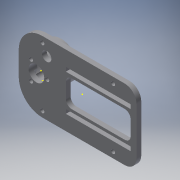
# Autodesk Inventor part: Slip_Plate_2bearing
Saved by Autodesk Inventor 2016 (Build 200138000, 138)
## iProperties
Created: 2015-10-15
Part Number: Slip_Plate_2bearing
Material: Generic
Document SubType Name: Modeling
Designer: USER
Density: 1 g/cm^3
Appearance: Default
Mass: 21.5255 g
Surface Area: 145.686 cm^2
Volume: 21.5255 cm^3
Author: USER
Autodesk Inventor part; units mm, degrees
ref_plane "YZ Plane" through (0, 0, 0) normal (1, 0, 0) x (0, 1, 0)
ref_plane "XZ Plane" through (0, 0, 0) normal (0, 1, 0) x (-1, 0, 0)
ref_plane "XY Plane" through (0, 0, 0) normal (0, 0, 1) x (1, 0, 0)
sketch "Sketch1" plane through (0, 0, 0) normal (0, 1, 0) x (-1, 0, 0)
  line L0 (-50, 30) -> (50, 30)
  line L1 (50, 30) -> (50, -30)
  line L2 (50, -30) -> (-50, -30)
  line L3 (-50, -30) -> (-50, 30)
  line L4 (0, 0) -> (0, 16.4238) construction
  line L5 (0, 0) -> (26.4574, 0) construction
  dimension "d0" = 100
  dimension "d1" = 60
  constraints: 12 end point, 3 parallel, 2 perpendicular, 1 horizontal, 2 other
  measures "d0" distance of L0.start L0.end
  measures "d1" distance of L0.end L1.end
extrude "Extrusion1" add sketch "Sketch1" along normal blind 4
sketch "Sketch2" plane through (0, 4, 0) normal (0, 1, 0) x (1, 0, 0)
  line L0 (50, -30) -> (50, 30) projected
  line L1 (-10, 17.25) -> (45, 17.25)
  line L2 (45, 17.25) -> (45, 13.75)
  line L3 (45, 13.75) -> (-10, 13.75)
  line L4 (-10, 13.75) -> (-10, 17.25)
  line L5 (-10, -13.75) -> (45, -13.75)
  line L6 (45, -13.75) -> (45, -17.25)
  line L7 (45, -17.25) -> (-10, -17.25)
  line L8 (-10, -17.25) -> (-10, -13.75)
  line L9 (0, 0) -> (41.7, 0) construction
  line L10 (-10, 15.5) -> (45, 15.5) construction
  line L11 (-10, -15.5) -> (45, -15.5) construction
  dimension "d4" = 3.5
  dimension "d5" = 31
  dimension "d6" = 5
  dimension "d7" = 55
  constraints: 22 end point, 4 midpoint, 4 parallel, 3 perpendicular, 2 horizontal, 4 other
  measures "d4" distance between parallel lines of L1 L3
  measures "d5" distance between parallel lines of L10 L11
  measures "d6" distance between parallel lines of L0 L2
  measures "d7" distance of L1.start L1.end
extrude "Extrusion2" cut sketch "Sketch2" against normal through all
sketch "Sketch3" plane through (0, 4, 0) normal (0, 1, 0) x (1, 0, 0)
  line L0 (-50, 30) -> (-50, -30) projected
  circle A0 centre (-35, 0) radius 6.65
  circle A1 centre (-25.79, 0) radius 1.7
  circle A2 centre (-39.605, 7.9761) radius 1.7
  circle A3 centre (-39.605, -7.9761) radius 1.7
  line L1 (-35, 0) -> (0, 0) construction
  line L2 (-35, 0) -> (-41.2469, 10.8199) construction
  line L3 (-35, 0) -> (-41.9983, -12.1214) construction
  circle A4 centre (-35, 0) radius 9.21 construction
  dimension "d10" = 120
  dimension "d11" = 120
  dimension "d12" = 18.42
  dimension "d13" = 13.3
  dimension "d14" = 3.4
  dimension "d15" = 3.4
  dimension "d16" = 3.4
  dimension "d17" = 15
  constraints: 6 end point, 5 centre point, 3 point on circle, 3 point on line, 1 coincident, 1 perpendicular
  measures "d10" angle of L2 L1
  measures "d11" angle of L3 L1
  measures "d12" diameter of A4
  measures "d13" diameter of A0
  measures "d14" diameter of A2
  measures "d15" diameter of A1
  measures "d16" diameter of A3
  measures "d17" distance from line of L0 L1.start
extrude "Extrusion3" cut sketch "Sketch3" against normal through all
sketch "Sketch4" plane through (0, 0, 0) normal (0, -1, 0) x (1, 0, 0)
  circle A0 centre (-35, 0) radius 6.65 projected
  line L0 (-10, 11.35) -> (45, 11.35)
  line L1 (45, 11.35) -> (45, -11.35)
  line L2 (45, -11.35) -> (-10, -11.35)
  line L3 (-10, -11.35) -> (-10, 11.35)
  line L4 (0, 0) -> (34.3745, 0) construction
  dimension "d20" = 25
  dimension "d21" = 55
  dimension "d22" = 22.7
  constraints: 10 end point, 2 parallel, 2 perpendicular, 1 horizontal, 1 other
  measures "d20" distance from line of L3 A0.centre
  measures "d21" distance of L0.start L0.end
  measures "d22" distance of L0.end L1.end
extrude "Extrusion4" cut sketch "Sketch4" against normal through all contours L0 L1 L2 L3
fillet "Fillet1" radius 10 2 edges at (50, 2, -30) (50, 2, 30)
fillet "Fillet2" radius 20 2 edges at (-50, 2, -30) (-50, 2, 30)
sketch "Sketch5" plane through (0, 0, 0) normal (0, -1, 0) x (1, 0, 0)
  line L0 (-50, 10) -> (-50, -10) projected
  line L1 (50, -20) -> (50, 20) projected
  line L2 (40, 30) -> (-30, 30) projected
  line L3 (-32.9422, 25) -> (22.0212, 25) construction
  line L4 (-20.947, -25) -> (23.6325, -25) construction
  line L5 (0, 0) -> (19.8728, 0) construction
  circle A0 centre (30, 25) radius 1.75
  circle A1 centre (-30, 25) radius 1.75
  circle A2 centre (-30, -25) radius 1.75
  circle A3 centre (30, -25) radius 1.75
  dimension "d27" = 5
  dimension "d28" = 3.5
  dimension "d29" = 3.5
  dimension "d30" = 20
  dimension "d31" = 20
  constraints: 6 end point, 4 centre point, 4 point on line, 3 parallel, 3 other
  measures "d27" distance between parallel lines of L2 L3
  measures "d28" diameter of A0
  measures "d29" diameter of A1
  measures "d30" distance from line of L0 A1.centre
  measures "d31" distance from line of L1 A0.centre
extrude "Extrusion5" cut sketch "Sketch5" against normal through all
fillet "Fillet3" radius 5 4 edges at (-10, 2, 11.35) (45, 2, 11.35) (45, 2, -11.35) (-10, 2, -11.35)
sketch "Sketch6" plane through (0, 4, 0) normal (0, 1, 0) x (1, 0, 0)
  circle A0 centre (-35, 0) radius 6.65 projected
  circle A1 centre (-35, 0) radius 11
  circle A2 centre (-35, 0) radius 6.65
  circle A3 centre (-35, 0) radius 15
  arc A4 (-24.3217, -2.6407) -> (-24.4212, 3.0147) centre (-26.9384, 0.1419) ccw
  arc A5 (-43.0674, -7.4777) -> (-37.985, -10.5872) centre (-39.1841, -6.8388) ccw
  arc A6 (-38.3451, 10.479) -> (-42.7646, 7.7917) centre (-39.7175, 7.7583) ccw
  point P0 (0, 0)
  dimension "d35" = 22
  constraints: 12 point on circle, 6 centre point, 3 coincident
  measures "d35" diameter of A1
extrude "Extrusion6" add sketch "Sketch6" along normal blind 17 contours A3
sketch "Sketch7" plane through (0, 4, 0) normal (0, 1, 0) x (1, 0, 0)
  point P0 (0, 0)
sketch "Sketch8" plane through (0, 4, 0) normal (0, 1, 0) x (1, 0, 0)
  point P0 (0, 0)
sketch "Sketch11" plane through (0, 4, 0) normal (0, 1, 0) x (1, 0, 0)
  arc A0 (-24.4212, 3.0147) -> (-38.3451, 10.479) centre (-35, 0) ccw projected
  line L0 (-38.3451, 10.479) -> (-34.5693, 6.636)
  line L1 (-24.4212, 3.0147) -> (-29.64, 3.9361)
  arc A1 (-29.64, 3.9361) -> (-34.5693, 6.636) centre (-35, 0) ccw
  arc A2 (-24.3217, -2.6407) -> (-24.4212, 3.0147) centre (-26.9384, 0.1419) ccw projected
  arc A3 (-24.4212, 3.0147) -> (-38.3451, 10.479) centre (-35, 0) ccw
  point P0 (0, 0)
  constraints: 4 end point, 4 point on circle, 2 centre point, 2 concentric
extrude "Extrusion9" add sketch "Sketch11" along normal blind 3
sketch "Sketch12" plane through (0, 4, 0) normal (0, 1, 0) x (1, 0, 0)
  line L0 (-43.0674, -7.4777) -> (-41.2773, -2.1949)
  arc A0 (-34.5693, 6.636) -> (-29.64, 3.9361) centre (-35, 0) ccw projected
  arc A1 (-42.7646, 7.7917) -> (-43.0674, -7.4777) centre (-35, 0) ccw projected
  line L1 (-42.7646, 7.7917) -> (-41.0562, 2.7469)
  arc A2 (-41.0562, 2.7469) -> (-41.2773, -2.1949) centre (-35, 0) ccw
  arc A3 (-38.3451, 10.479) -> (-42.7646, 7.7917) centre (-39.7175, 7.7583) ccw projected
  arc A4 (-42.7646, 7.7917) -> (-43.0674, -7.4777) centre (-35, 0) ccw
  point P0 (0, 0)
  constraints: 6 point on circle, 4 end point, 2 centre point, 2 concentric
extrude "Extrusion10" add sketch "Sketch12" along normal blind 3
sketch "Sketch13" plane through (0, 4, 0) normal (0, 1, 0) x (1, 0, 0)
  arc A0 (-24.3217, -2.6407) -> (-24.4212, 3.0147) centre (-26.9384, 0.1419) ccw projected
  line L0 (-24.3217, -2.6407) -> (-29.3899, -3.5706)
  arc A1 (-41.2773, -2.1949) -> (-29.64, 3.9361) centre (-35, 0) ccw projected
  arc A2 (-37.985, -10.5872) -> (-24.3217, -2.6407) centre (-35, 0) ccw projected
  line L1 (-37.985, -10.5872) -> (-34.3481, -6.618)
  arc A3 (-34.3481, -6.618) -> (-29.3899, -3.5706) centre (-35, 0) ccw
  arc A4 (-37.985, -10.5872) -> (-24.3217, -2.6407) centre (-35, 0) ccw
  point P0 (0, 0)
  constraints: 6 point on circle, 4 end point, 3 concentric, 2 centre point
extrude "Extrusion11" add sketch "Sketch13" along normal blind 3
sketch "Sketch14" plane through (0, 4, 0) normal (0, 1, 0) x (1, 0, 0)
  arc A0 (-29.64, 3.9361) -> (-34.5693, 6.636) centre (-35, 0) ccw projected
  point P0 (0, 0)
sketch "Sketch15" plane through (0, 21, 0) normal (0, 1, 0) x (1, 0, 0)
  point P0 (0, 0)
sketch "Sketch16" plane through (0, 21, 0) normal (0, 1, 0) x (1, 0, 0)
  arc A0 (-42.7646, 7.7917) -> (-43.0674, -7.4777) centre (-35, 0) ccw projected
  circle A1 centre (-35, 0) radius 6.65 projected
  circle A2 centre (-35, 0) radius 11.25
  circle A3 centre (-35, 0) radius 11
  point P0 (0, 0)
  dimension "d53" = 22.5
  dimension "d54" = 22
  constraints: 2 centre point, 2 coincident
  measures "d53" diameter of A2
  measures "d54" diameter of A3
extrude "Extrusion12" cut sketch "Sketch16" against normal blind 14 contours A2
sketch "Sketch17" plane through (0, 4, 0) normal (0, 1, 0) x (1, 0, 0)
  circle A0 centre (-26.2915, -16.8922) radius 4.0048
  circle A1 centre (-35, 0) radius 15 projected
  point P0 (0, 0)
  point P1 (-50, 0)
  constraints: 1 centre point, 1 horizontal alignment, 1 other
extrude "Extrusion13" cut sketch "Sketch17" against normal blind 4 contours A0
body "Solid1"
